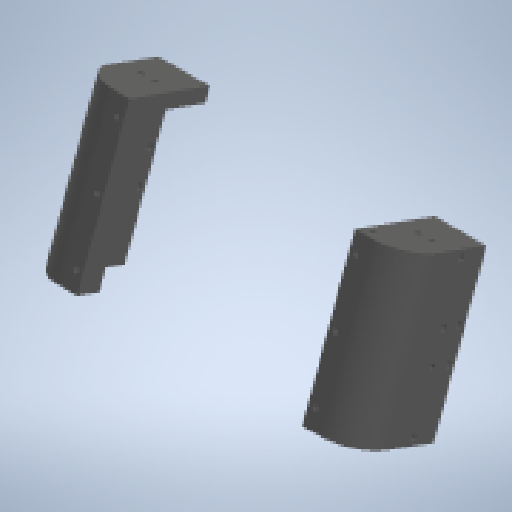
# Autodesk Inventor part: chest_cover_side
Saved by Autodesk Inventor 2024.1 (Build 281209000, 209)
## iProperties
Created: 2024-02-14
Part Number: chest_cover_side
Material: 一般
Document SubType Name: Modeling
Designer: hibik
Density: 1 g/cm^3
Appearance: 既定
Author: hibik
Autodesk Inventor part; units mm, degrees
ref_plane "YZ Plane" through (0, 0, 0) normal (1, 0, 0) x (0, 1, 0)
ref_plane "XZ Plane" through (0, 0, 0) normal (0, 1, 0) x (-1, 0, 0)
sketch "スケッチ1" plane through (0, 0, 0) normal (1, 0, 0) x (0, 1, 0)
  line L0 (0, 0) -> (33, 0)
  line L1 (33, 0) -> (3.8603, 10.606)
  line L2 (3.8603, 10.606) -> (0, 0)
  line L3 (33, 0) -> (3.8603, 10.606)
  line L4 (3.8603, 10.606) -> (5.2283, 14.3648)
  line L5 (5.2283, 14.3648) -> (34.3681, 3.7588)
  line L6 (34.3681, 3.7588) -> (33, 0)
  line L7 (5.2283, 14.3648) -> (0, 12.011)
  line L8 (0, 12.011) -> (3.8603, 10.606)
  line L9 (0, 0) -> (0, 12.011)
  circle A0 centre (2, 10.7181) radius 0.8
  line L10 (34.3681, 3.7588) -> (42.9186, 27.2511)
  line L11 (42.9186, 27.2511) -> (8.15, 39.9058)
  line L12 (8.15, 39.9058) -> (-0.4005, 16.4135)
  line L13 (-0.4005, 16.4135) -> (34.3681, 3.7588)
  line L14 (-0.4005, 16.4135) -> (8.15, 39.9058)
  line L15 (8.15, 39.9058) -> (50.4361, 24.5149)
  line L16 (50.4361, 24.5149) -> (41.8856, 1.0226)
  line L17 (41.8856, 1.0226) -> (-0.4005, 16.4135)
  line L18 (8.15, 39.9058) -> (-1.9502, 12.1558)
  line L19 (-1.9502, 12.1558) -> (2, 10.7181)
  line L20 (42.5697, 2.902) -> (0.2835, 18.2929)
  point P0 (0.2835, 18.2929)
  point P1 (-0.4005, 16.4135)
  point P2 (35.0521, 5.6382)
  point P3 (42.9186, 27.2511)
  dimension "d0" = 33
  dimension "d1" = 20
  dimension "d2" = 4
  dimension "d3" = 1.6
  dimension "d4" = 2
  dimension "d5" = 2
  dimension "d6" = 25
  dimension "d7" = 37
  dimension "d8" = 45
  dimension "d10" = 2
  constraints: 42 end point, 7 parallel, 6 perpendicular, 3 collinear, 3 point on line, 1 centre point, 1 coincident, 1 horizontal, 1 vertical
  measures "d0" distance of L0.start L0.end
  measures "d1" angle of L0 L1
  measures "d2" distance of L1.end L4.end
  measures "d3" diameter of A0
  measures "d4" distance from line of L7 L19.end
  measures "d5" distance from line of L9 L19.end
  measures "d6" distance between parallel lines of L5 L11
  measures "d7" distance between parallel lines of L12 L10
  measures "d8" distance between parallel lines of L12 L16
  measures "d10" distance between parallel lines of L17 L20
extrude "押し出し1" add sketch "スケッチ1" along normal blind 15 contours L5 L13 L12 L20 L10 | L10 L20 L16 L17 | L20 L12 L11 L10 | L10 L15 L16 L20
sketch "スケッチ2" plane through (0, 3.4515, 41.6159) normal (0, 0.3420201, 0.9396926) x (1, 0, 0)
  line L0 (0, 50) -> (5.2556, 50)
  line L1 (0, 0) -> (0, 50)
  circle A0 centre (2, 45) radius 0.8
  circle A1 centre (2, 10) radius 0.8
  circle A2 centre (2, 27.5) radius 0.8
  line L2 (0, 50) -> (4, 50)
  line L3 (4, 50) -> (4, 5)
  line L4 (4, 5) -> (0, 5)
  line L5 (0, 5) -> (0, 50)
  line L6 (0, 50) -> (0, 5) projected
  dimension "d13" = 1.6
  dimension "d14" = 1.6
  dimension "d15" = 1.6
  dimension "d18" = 5
  dimension "d19" = 17.5
  dimension "d21" = 17.5
  dimension "d22" = 2
  dimension "d23" = 4
  dimension "d30" = 5
  constraints: 12 end point, 3 centre point, 2 horizontal, 2 parallel, 2 vertical alignment, 1 collinear, 1 perpendicular
  measures "d13" diameter of A0
  measures "d14" diameter of A1
  measures "d15" diameter of A2
  measures "d18" distance from line of L4 A1.centre
  measures "d19" distance of A2.centre A0.centre
  measures "d21" distance of A2.centre A1.centre
  measures "d22" distance from line of A0.centre L5
  measures "d23" distance between parallel lines of L6 L3
  measures "d30" distance from line of L0 A0.centre
extrude "押し出し2" cut sketch "スケッチ2" against normal through all contours A0 | A1 | A2
ref_plane "作業平面1" through (-33, 0, 0) normal (-1, 0, 0) x (0, 0, 1)
mirror "ミラー1" about plane through (-33, 0, 0) normal (-1, 0, 0)
sketch "スケッチ4" plane through (-81, 2.3356, 23.9311) normal (-1, 0, 0) x (0, 0.3420201, 0.9396926)
  circle A0 centre (-6, 18) radius 0.8 projected
  circle A1 centre (-1, 18) radius 0.8 projected
  circle A2 centre (-1, 2) radius 0.8 projected
  line L0 (-8, 45) -> (17, 45) projected
  line L1 (-8, 0) -> (-8, 45) projected
  line L2 (17, 0) -> (-8, 0) projected
  line L3 (-8, 22.5) -> (0, 22.5)
  circle A3 centre (-6, 27) radius 0.8
  circle A4 centre (-1, 27) radius 0.8
  circle A5 centre (-1, 43) radius 0.8
  line L4 (17, 45) -> (17, 0) projected
  point P0 (-23.2867, 5.9901)
  constraints: 3 centre point, 3 symmetric about line, 2 end point, 1 midpoint, 3 other
extrude "押し出し4" cut sketch "スケッチ4" against normal through all contours A0 | A1 | A2 | A3 | A4 | A5
sketch "スケッチ5" plane through (-81, 41.8856, 1.0226) normal (0, 0.9396926, -0.3420201) x (1, 0, 0)
  circle A0 centre (83.3679, -22) radius 0.8 projected
  circle A1 centre (86.5298, -11.2421) radius 0.8 projected
  circle A2 centre (90.5298, -11.2421) radius 0.8 projected
  circle A3 centre (12.6321, -22) radius 0.8 projected
  circle A4 centre (9.4702, -11.2421) radius 0.8 projected
  circle A5 centre (5.4702, -11.2421) radius 0.8 projected
  point P0 (81, 15.2867)
extrude "押し出し5" cut sketch "スケッチ5" against normal through all
fillet "フィレット1" radius 10 2 edges at (-81, 29.293, 32.2104) (15, 29.293, 32.2104)
sketch "スケッチ6" plane through (-81, 41.8856, 1.0226) normal (0, 0.9396926, -0.3420201) x (1, 0, 0)
  line L0 (81, 0) -> (96, 0) projected
  line L1 (90.5, 0) -> (5.5, 0)
  line L2 (5.5, 0) -> (5.5, -18)
  line L3 (5.5, -18) -> (90.5, -18)
  line L4 (90.5, -18) -> (90.5, 0)
  line L5 (81, -25) -> (81, 0) projected
  line L6 (15, -25) -> (0, -25) projected
  line L7 (81, -25) -> (15, -25) construction
  point P0 (81, 15.2867)
  point P1 (81, -22.6101)
  point P2 (11, -25)
  point P3 (48, -25)
  point P4 (48, -18)
  dimension "d40" = 18
  dimension "d41" = 85
  constraints: 10 end point, 2 horizontal, 2 midpoint, 2 parallel, 1 perpendicular, 1 point on line, 1 vertical alignment
  measures "d40" distance of L3.end L1.start
  measures "d41" distance of L2.end L3.end
extrude "押し出し6" cut sketch "スケッチ6" against normal through all
sketch "スケッチ7" plane through (0, 50.4361, 24.5149) normal (0, 0.9396926, -0.3420201) x (1, 0, 0)
  circle A0 centre (2.3679, 3) radius 0.8 projected
  line L0 (9.5, 25) -> (9.5, 14.5574) projected
  arc A1 (9.5, 12.9585) -> (9.5, 14.5574) centre (9.5298, 13.7579) ccw projected
  line L1 (9.5, 12.9585) -> (9.5, 7) projected
  line L2 (9.5, 7) -> (0, 7) projected
  line L3 (0, 7) -> (0, 0) projected
  line L4 (0, 0) -> (5, 0) projected
  arc A2 (5, 0) -> (15, 10) centre (5, 10) ccw projected
  line L5 (15, 25) -> (15, 10) projected
  line L6 (9.5, 25) -> (15, 25) projected
  line L7 (-75.5, 14.5574) -> (-75.5, 25) projected
  line L8 (-75.5, 25) -> (-81, 25) projected
  line L9 (-81, 25) -> (-81, 10) projected
  arc A3 (-81, 10) -> (-71, 0) centre (-71, 10) ccw projected
  line L10 (-66, 0) -> (-71, 0) projected
  line L11 (-66, 7) -> (-66, 0) projected
  line L12 (-66, 7) -> (-75.5, 7) projected
  line L13 (-75.5, 7) -> (-75.5, 12.9585) projected
  arc A4 (-75.5, 14.5574) -> (-75.5, 12.9585) centre (-75.5298, 13.7579) ccw projected
  circle A5 centre (-68.3679, 3) radius 0.8 projected
  line L14 (15, 0) -> (0, 0)
  line L15 (0, 0) -> (0, 25)
  line L16 (0, 25) -> (15, 25)
  line L17 (15, 25) -> (15, 0)
  line L18 (-66, 0) -> (-81, 0)
  line L19 (-81, 0) -> (-81, 25)
  line L20 (-81, 25) -> (-66, 25)
  line L21 (-66, 25) -> (-66, 0)
  line L22 (15, 25) -> (15, 10) projected
  point P0 (0, 40.2867)
  constraints: 16 end point, 6 collinear, 4 parallel, 2 horizontal, 2 perpendicular, 1 point on line
extrude "押し出し7" add sketch "スケッチ7" against normal blind 4 contours L0 A1 L1 L2 L15 L16 | A4 L13 L12 L11 L10 A3 L9 L8 L7 | L7 L20 L21 L12 L13 A4 | A5
sketch "スケッチ8" plane through (0, 41.8856, 1.0226) normal (0, 0.9396926, -0.3420201) x (1, 0, 0)
  circle A0 centre (9.5298, -11.2421) radius 0.8 projected
  circle A1 centre (5.5298, -11.2421) radius 0.8 projected
  circle A2 centre (-71.5298, -11.2421) radius 0.8 projected
  circle A3 centre (9.5298, -11.2421) radius 0.8 projected
  circle A4 centre (-68.3679, -22) radius 0.8 projected
  circle A5 centre (5.5298, -11.2421) radius 0.8 projected
  circle A6 centre (-75.5298, -11.2421) radius 0.8 projected
  circle A7 centre (-71.5298, -11.2421) radius 0.8 projected
  circle A8 centre (2.3679, -22) radius 0.8 projected
  arc A9 (-16.0839, 0) -> (-19.042, -2.5) centre (-16.0839, -3) ccw projected
  arc A10 (-22, -5) -> (-19.042, -2.5) centre (-22, -2) ccw projected
  line L0 (-44, -5) -> (-22, -5) projected
  arc A11 (-46.958, -2.5) -> (-44, -5) centre (-44, -2) ccw projected
  arc A12 (-46.958, -2.5) -> (-49.9161, 0) centre (-49.9161, -3) ccw projected
  line L1 (-78, 0) -> (-49.9161, 0) projected
  arc A13 (-78, 0) -> (-81, -3) centre (-78, -3) ccw projected
  line L2 (-81, -15) -> (-81, -3) projected
  arc A14 (-81, -15) -> (-71, -25) centre (-71, -15) ccw projected
  line L3 (-71, -25) -> (5, -25) projected
  arc A15 (5, -25) -> (15, -15) centre (5, -15) ccw projected
  line L4 (15, -3) -> (15, -15) projected
  arc A16 (15, -3) -> (12, 0) centre (12, -3) ccw projected
  line L5 (-16.0839, 0) -> (12, 0) projected
  arc A17 (-46.8433, -9.5397) -> (-48.6909, -6.7698) centre (-49.8433, -9.5397) ccw projected
  line L6 (-46.8433, -9.5397) -> (-46.8433, -20) projected
  arc A18 (-49.8433, -23) -> (-46.8433, -20) centre (-49.8433, -20) ccw projected
  line L7 (-49.8433, -23) -> (-51.6865, -23) projected
  arc A19 (-54.6865, -20) -> (-51.6865, -23) centre (-51.6865, -20) ccw projected
  line L8 (-54.6865, -20) -> (-54.6865, -8.3352) projected
  arc A20 (-49.6125, -6.1676) -> (-54.6865, -8.3352) centre (-51.6865, -8.3352) ccw projected
  arc A21 (-49.6125, -6.1676) -> (-48.6909, -6.7698) centre (-47.5384, -4) ccw projected
  line L9 (-38, -23) -> (-39.8433, -23) projected
  arc A22 (-42.8433, -20) -> (-39.8433, -23) centre (-39.8433, -20) ccw projected
  line L10 (-42.8433, -20) -> (-42.8433, -10) projected
  arc A23 (-39.8433, -7) -> (-42.8433, -10) centre (-39.8433, -10) ccw projected
  line L11 (-39.8433, -7) -> (-38, -7) projected
  arc A24 (-35, -10) -> (-38, -7) centre (-38, -10) ccw projected
  line L12 (-35, -10) -> (-35, -20) projected
  arc A25 (-38, -23) -> (-35, -20) centre (-38, -20) ccw projected
  line L13 (0.5298, -5) -> (0.5298, -20) projected
  arc A26 (-2.4702, -23) -> (0.5298, -20) centre (-2.4702, -20) ccw projected
  line L14 (-2.4702, -23) -> (-4.3135, -23) projected
  arc A27 (-7.3135, -20) -> (-4.3135, -23) centre (-4.3135, -20) ccw projected
  line L15 (-7.3135, -20) -> (-7.3135, -5) projected
  arc A28 (-4.3135, -2) -> (-7.3135, -5) centre (-4.3135, -5) ccw projected
  line L16 (-4.3135, -2) -> (-2.4702, -2) projected
  arc A29 (0.5298, -5) -> (-2.4702, -2) centre (-2.4702, -5) ccw projected
  line L17 (-66.5298, -20) -> (-66.5298, -5) projected
  arc A30 (-63.5298, -2) -> (-66.5298, -5) centre (-63.5298, -5) ccw projected
  line L18 (-63.5298, -2) -> (-61.6865, -2) projected
  arc A31 (-58.6865, -5) -> (-61.6865, -2) centre (-61.6865, -5) ccw projected
  line L19 (-58.6865, -5) -> (-58.6865, -20) projected
  arc A32 (-61.6865, -23) -> (-58.6865, -20) centre (-61.6865, -20) ccw projected
  line L20 (-61.6865, -23) -> (-63.5298, -23) projected
  arc A33 (-66.5298, -20) -> (-63.5298, -23) centre (-63.5298, -20) ccw projected
  line L21 (4.5298, -6.6595) -> (4.5298, -5) projected
  arc A34 (7.5298, -2) -> (4.5298, -5) centre (7.5298, -5) ccw projected
  line L22 (7.5298, -2) -> (8, -2) projected
  arc A35 (11, -5) -> (8, -2) centre (8, -5) ccw projected
  line L23 (11, -5) -> (11, -5.9328) projected
  arc A36 (10.5187, -7.5626) -> (11, -5.9328) centre (8, -5.9328) ccw projected
  line L24 (10.5187, -7.5626) -> (10.0485, -8.2893) projected
  arc A37 (4.5298, -6.6595) -> (10.0485, -8.2893) centre (7.5298, -6.6595) ccw projected
  line L25 (-70.5298, -5) -> (-70.5298, -6.6595) projected
  arc A38 (-76.0485, -8.2893) -> (-70.5298, -6.6595) centre (-73.5298, -6.6595) ccw projected
  line L26 (-76.0485, -8.2893) -> (-76.5187, -7.5626) projected
  arc A39 (-77, -5.9328) -> (-76.5187, -7.5626) centre (-74, -5.9328) ccw projected
  line L27 (-77, -5.9328) -> (-77, -5) projected
  arc A40 (-74, -2) -> (-77, -5) centre (-74, -5) ccw projected
  line L28 (-74, -2) -> (-73.5298, -2) projected
  arc A41 (-70.5298, -5) -> (-73.5298, -2) centre (-73.5298, -5) ccw projected
  arc A42 (-17.3091, -6.7698) -> (-16.3875, -6.1676) centre (-18.4616, -4) ccw projected
  arc A43 (-11.3135, -8.3352) -> (-16.3875, -6.1676) centre (-14.3135, -8.3352) ccw projected
  line L29 (-11.3135, -8.3352) -> (-11.3135, -20) projected
  arc A44 (-14.3135, -23) -> (-11.3135, -20) centre (-14.3135, -20) ccw projected
  line L30 (-14.3135, -23) -> (-16.1567, -23) projected
  arc A45 (-19.1567, -20) -> (-16.1567, -23) centre (-16.1567, -20) ccw projected
  line L31 (-19.1567, -20) -> (-19.1567, -9.5397) projected
  arc A46 (-17.3091, -6.7698) -> (-19.1567, -9.5397) centre (-16.1567, -9.5397) ccw projected
  line L32 (-26.1567, -23) -> (-28, -23) projected
  arc A47 (-31, -20) -> (-28, -23) centre (-28, -20) ccw projected
  line L33 (-31, -20) -> (-31, -10) projected
  arc A48 (-28, -7) -> (-31, -10) centre (-28, -10) ccw projected
  line L34 (-28, -7) -> (-26.1567, -7) projected
  arc A49 (-23.1567, -10) -> (-26.1567, -7) centre (-26.1567, -10) ccw projected
  line L35 (-23.1567, -10) -> (-23.1567, -20) projected
  arc A50 (-26.1567, -23) -> (-23.1567, -20) centre (-26.1567, -20) ccw projected
  point P0 (0, 15.2867)
extrude "押し出し8" cut sketch "スケッチ8" against normal through all contours A0 | A1 | A2 | A6
equation "\"d5\" = d4"
equation "\"d19\" = d21"
